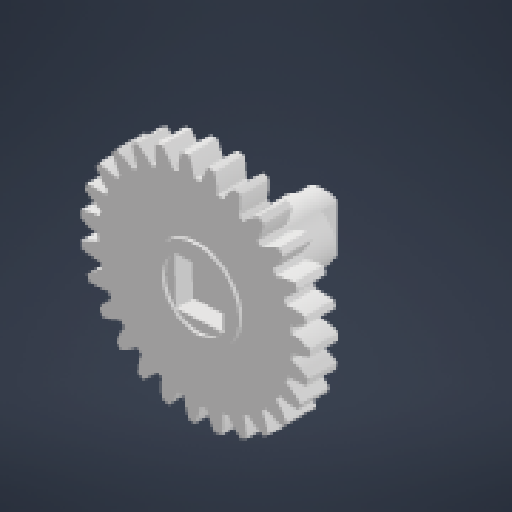
# Autodesk Inventor part: central axel
Saved by Autodesk Inventor 2026 (Build 300175050, 175E)
## iProperties
Created: 2026-03-26
Part Number: central axel
Material: Generic
Document SubType Name: Modeling
Designer: sniel
Density: 1 g/cm^3
Appearance: Default
Author: sniel
Autodesk Inventor part; units mm, degrees
ref_plane "YZ Plane" through (0, 0, 0) normal (1, 0, 0) x (0, 1, 0)
ref_plane "XZ Plane" through (0, 0, 0) normal (0, 1, 0) x (-1, 0, 0)
sketch "Sketch1" plane through (0, 0, 0) normal (0, 0, 1) x (1, 0, 0)
  arc A0 (-2.5, -4.3301) -> (2.5, -4.3301) centre (0, 0) ccw
  line L0 (2.5, 4.3301) -> (2.5, -4.3301)
  arc A1 (2.5, 4.3301) -> (-2.5, 4.3301) centre (0, 0) ccw
  line L1 (-2.5, -4.3301) -> (-2.5, 4.3301)
  line L2 (0, -5) -> (0, -4.75)
  circle A2 centre (0, 0) radius 4.75
  line L3 (-2.5, 0) -> (-2.4, 0)
  line L4 (2.5, 0) -> (2.4, 0)
  line L5 (-2.4, 0) -> (-2.4, -4.3863)
  line L6 (2.4, 0) -> (2.4, -4.3863)
  line L7 (2.4, 0) -> (2.4, 4.3863)
  line L8 (-2.4, 0) -> (-2.4, 4.3863)
  point P0 (0, 0)
  point P1 (-2.4, 4.0991)
  point P2 (-2.4, -4.0991)
  point P3 (2.4, -4.0991)
  point P4 (2.4, 4.0991)
  dimension "d0" = 0.25
  dimension "d1" = 0.1
  dimension "d2" = 0.1
  constraints: 18 end point, 9 point on circle, 4 vertical, 2 centre point, 2 horizontal, 2 midpoint, 1 coincident, 3 other
  measures "d0" distance of L2.start L2.end
  measures "d1" distance of L3.start L3.end
  measures "d2" distance of L4.start L4.end
extrude "Extrusion1" add sketch "Sketch1" along normal blind 3 contours L5 L8 A2 L7 L6
ref_plane "Work Plane1" through (-110.4204, -110.4204, 21.5411) normal (0, 0, -1) x (-0.0508, 0.9987, 0)
sketch "Sketch2" plane through (0, 0, 3) normal (0, 0, 1) x (1, 0, 0)
  circle A0 centre (0, 0) radius 5
  dimension "d5" = 10
  constraints: 1 centre point, 1 coincident
  measures "d5" diameter of A0
extrude "Extrusion2" add sketch "Sketch2" along normal up to surface (18.5411 mm away)
sketch "Sketch3" plane through (0, 0, 21.5411) normal (0, 0, 1) x (1, 0, 0)
  arc A0 (-4.8284, 16.7732) -> (-6.3222, 18.8577) centre (-16.1161, 10.2619) ccw
  arc A1 (-6.3222, 18.8577) -> (-7.4127, 18.4955) centre (-0.6419, -0.0624) ccw
  arc A2 (-7.4127, 18.4955) -> (-7.264, 15.2567) centre (5.5779, 17.4691) ccw
  arc A3 (-7.264, 15.2567) -> (-8.1435, 14.8457) centre (-0.6419, -0.0624) ccw
  arc A4 (-8.1435, 14.8457) -> (-10.5324, 17.0378) centre (-18.0799, 6.415) ccw
  arc A5 (-10.5324, 17.0378) -> (-11.5099, 16.4338) centre (-0.6419, -0.0624) ccw
  arc A6 (-11.5099, 16.4338) -> (-10.6183, 13.3166) centre (1.3672, 18.4309) ccw
  arc A7 (-10.6183, 13.3166) -> (-11.3793, 12.7139) centre (-0.6419, -0.0624) ccw
  arc A8 (-11.3793, 12.7139) -> (-14.2093, 14.296) centre (-19.1036, 2.2189) ccw
  arc A9 (-14.2093, 14.296) -> (-15.0212, 13.4828) centre (-0.6419, -0.0624) ccw
  arc A10 (-15.0212, 13.4828) -> (-13.4348, 10.6552) centre (-2.9518, 18.3958) ccw
  arc A11 (-13.4348, 10.6552) -> (-14.0363, 9.8933) centre (-0.6419, -0.0624) ccw
  arc A12 (-14.0363, 9.8933) -> (-17.1549, 10.7801) centre (-19.1321, -2.1002) ccw
  arc A13 (-17.1549, 10.7801) -> (-17.7574, 9.8016) centre (-0.6419, -0.0624) ccw
  arc A14 (-17.7574, 9.8016) -> (-15.5616, 7.4161) centre (-7.1463, 17.3655) ccw
  arc A15 (-15.5616, 7.4161) -> (-15.9712, 6.5359) centre (-0.6419, -0.0624) ccw
  arc A16 (-15.9712, 6.5359) -> (-19.2102, 6.6796) centre (-18.1638, -6.3094) ccw
  arc A17 (-19.2102, 6.6796) -> (-19.5708, 5.5886) centre (-0.6419, -0.0624) ccw
  arc A18 (-19.5708, 5.5886) -> (-16.8841, 3.7738) centre (-10.9901, 15.3958) ccw
  arc A19 (-16.8841, 3.7738) -> (-17.0797, 2.8229) centre (-0.6419, -0.0624) ccw
  arc A20 (-17.0797, 2.8229) -> (-20.2645, 2.2158) centre (-16.2508, -10.1818) ccw
  arc A21 (-20.2645, 2.2158) -> (-20.3638, 1.0709) centre (-0.6419, -0.0624) ccw
  arc A22 (-20.3638, 1.0709) -> (-17.331, -0.0753) centre (-14.2761, 12.5926) ccw
  arc A23 (-17.331, -0.0753) -> (-17.302, -1.0457) centre (-0.6419, -0.0624) ccw
  arc A24 (-17.302, -1.0457) -> (-20.261, -2.3709) centre (-13.4964, -13.5087) ccw
  arc A25 (-20.261, -2.3709) -> (-20.0936, -3.5078) centre (-0.6419, -0.0624) ccw
  arc A26 (-20.0936, -3.5078) -> (-16.8782, -3.9237) centre (-16.827, 9.1072) ccw
  arc A27 (-16.8782, -3.9237) -> (-16.6262, -4.8613) centre (-0.6419, -0.0624) ccw
  arc A28 (-16.6262, -4.8613) -> (-19.1998, -6.8332) centre (-10.049, -16.1107) ccw
  arc A29 (-19.1998, -6.8332) -> (-18.7747, -7.9008) centre (-0.6419, -0.0624) ccw
  arc A30 (-18.7747, -7.9008) -> (-15.55, -7.564) centre (-18.5054, 5.1275) ccw
  arc A31 (-15.55, -7.564) -> (-15.0886, -8.4181) centre (-0.6419, -0.0624) ccw
  arc A32 (-15.0886, -8.4181) -> (-17.1381, -10.9304) centre (-6.0944, -17.8475) ccw
  arc A33 (-17.1381, -10.9304) -> (-16.4783, -11.8712) centre (-0.6419, -0.0624) ccw
  arc A34 (-16.4783, -11.8712) -> (-13.4182, -10.7998) centre (-19.2208, 0.868) ccw
  arc A35 (-13.4182, -10.7998) -> (-12.7722, -11.5246) centre (-0.6419, -0.0624) ccw
  arc A36 (-12.7722, -11.5246) -> (-14.1871, -14.4418) centre (-1.8459, -18.6256) ccw
  arc A37 (-14.1871, -14.4418) -> (-13.3281, -15.205) centre (-0.6419, -0.0624) ccw
  arc A38 (-13.3281, -15.205) -> (-10.5976, -13.4568) centre (-18.9346, -3.4416) ccw
  arc A39 (-10.5976, -13.4568) -> (-9.8019, -14.013) centre (-0.6419, -0.0624) ccw
  arc A40 (-9.8019, -14.013) -> (-10.5059, -17.1779) centre (2.4675, -18.4029) ccw
  arc A41 (-10.5059, -17.1779) -> (-9.494, -17.7225) centre (-0.6419, -0.0624) ccw
  arc A42 (-9.494, -17.7225) -> (-7.2402, -15.3917) centre (-17.6622, -7.5691) ccw
  arc A43 (-7.2402, -15.3917) -> (-6.3378, -15.7494) centre (-0.6419, -0.0624) ccw
  arc A44 (-6.3378, -15.7494) -> (-6.2929, -18.9913) centre (6.6133, -17.1914) ccw
  arc A45 (-6.2929, -18.9913) -> (-5.1827, -19.2879) centre (-0.6419, -0.0624) ccw
  arc A46 (-5.1827, -19.2879) -> (-3.5272, -16.5002) centre (-15.4722, -11.2919) ccw
  arc A47 (-3.5272, -16.5002) -> (-2.5666, -16.6401) centre (-0.6419, -0.0624) ccw
  arc A48 (-2.5666, -16.6401) -> (-1.7752, -19.7843) centre (10.3679, -15.0565) ccw
  arc A49 (-1.7752, -19.7843) -> (-0.6266, -19.8168) centre (-0.6419, -0.0624) ccw
  arc A50 (-0.6266, -19.8168) -> (0.3414, -16.7225) centre (-12.4828, -14.4093) ccw
  arc A51 (0.3414, -16.7225) -> (1.3084, -16.6371) centre (-0.6419, -0.0624) ccw
  arc A52 (1.3084, -16.6371) -> (2.8035, -19.5141) centre (13.5291, -12.1133) ccw
  arc A53 (2.8035, -19.5141) -> (3.9287, -19.2808) centre (-0.6419, -0.0624) ccw
  arc A54 (3.9287, -19.2808) -> (4.157, -16.0467) centre (-8.8549, -16.7533) ccw
  arc A55 (4.157, -16.0467) -> (5.0782, -15.7406) centre (-0.6419, -0.0624) ccw
  arc A56 (5.0782, -15.7406) -> (7.1965, -18.1952) centre (15.9262, -8.5204) ccw
  arc A57 (7.1965, -18.1952) -> (8.2375, -17.7087) centre (-0.6419, -0.0624) ccw
  arc A58 (8.2375, -17.7087) -> (7.7138, -14.5091) centre (-4.7844, -18.1975) ccw
  arc A59 (7.7138, -14.5091) -> (8.5397, -13.9988) centre (-0.6419, -0.0624) ccw
  arc A60 (8.5397, -13.9988) -> (11.1669, -15.8988) centre (17.4302, -4.4716) ccw
  arc A61 (11.1669, -15.8988) -> (12.0677, -15.1853) centre (-0.6419, -0.0624) ccw
  arc A62 (12.0677, -15.1853) -> (10.8202, -12.1927) centre (-0.4905, -18.664) ccw
  arc A63 (10.8202, -12.1927) -> (11.5062, -11.5058) centre (-0.6419, -0.0624) ccw
  arc A64 (11.5062, -11.5058) -> (14.5007, -12.7486) centre (17.9599, -0.185) ccw
  arc A65 (14.5007, -12.7486) -> (15.2127, -11.8467) centre (-0.6419, -0.0624) ccw
  arc A66 (15.2127, -11.8467) -> (13.3087, -9.2224) centre (3.7952, -18.1276) ccw
  arc A67 (13.3087, -9.2224) -> (13.8177, -8.3958) centre (-0.6419, -0.0624) ccw
  arc A68 (13.8177, -8.3958) -> (17.0182, -8.9145) centre (17.4867, 4.1081) ccw
  arc A69 (17.0182, -8.9145) -> (17.503, -7.8727) centre (-0.6419, -0.0624) ccw
  arc A70 (17.503, -7.8727) -> (15.0451, -5.7583) centre (7.8418, -16.6174) ccw
  arc A71 (15.0451, -5.7583) -> (15.3498, -4.8365) centre (-0.6419, -0.0624) ccw
  arc A72 (15.3498, -4.8365) -> (18.5836, -4.6032) centre (16.0363, 8.1765) ccw
  arc A73 (18.5836, -4.6032) -> (18.8151, -3.4777) centre (-0.6419, -0.0624) ccw
  arc A74 (18.8151, -3.4777) -> (15.9358, -1.9871) centre (11.4309, -14.2147) ccw
  arc A75 (15.9358, -1.9871) -> (16.0197, -1.0199) centre (-0.6419, -0.0624) ccw
  arc A76 (16.0197, -1.0199) -> (19.1125, -0.0471) centre (13.6867, 11.8006) ccw
  arc A77 (19.1125, -0.0471) -> (19.0782, 1.1015) centre (-0.6419, -0.0624) ccw
  arc A78 (19.0782, 1.1015) -> (15.9328, 1.8879) centre (14.3693, -11.049) ccw
  arc A79 (15.9328, 1.8879) -> (15.7914, 2.8483) centre (-0.6419, -0.0624) ccw
  arc A80 (15.7914, 2.8483) -> (18.5765, 4.5082) centre (10.5647, 14.7853) ccw
  arc A81 (18.5765, 4.5082) -> (18.2783, 5.6179) centre (-0.6419, -0.0624) ccw
  arc A82 (18.2783, 5.6179) -> (15.0363, 5.6577) centre (16.4983, -7.2911) ccw
  arc A83 (15.0363, 5.6577) -> (14.6772, 6.5597) centre (-0.6419, -0.0624) ccw
  arc A84 (14.6772, 6.5597) -> (17.0044, 8.817) centre (6.8385, 16.9695) ccw
  arc A85 (17.0044, 8.817) -> (16.4583, 9.8281) centre (-0.6419, -0.0624) ccw
  arc A86 (16.4583, 9.8281) -> (13.2945, 9.1192) centre (17.7033, -3.1434) ccw
  arc A87 (13.2945, 9.1192) -> (12.7371, 9.914) centre (-0.6419, -0.0624) ccw
  arc A88 (12.7371, 9.914) -> (14.481, 12.6472) centre (2.709, 18.2355) ccw
  arc A89 (14.481, 12.6472) -> (13.7165, 13.505) centre (-0.6419, -0.0624) ccw
  arc A90 (13.7165, 13.505) -> (10.8014, 12.0857) centre (17.9194, 1.1703) ccw
  arc A91 (10.8014, 12.0857) -> (10.0757, 12.7305) centre (-0.6419, -0.0624) ccw
  arc A92 (10.0757, 12.7305) -> (11.1424, 15.7922) centre (-1.6011, 18.515) ccw
  arc A93 (11.1424, 15.7922) -> (10.2006, 16.4506) centre (-0.6419, -0.0624) ccw
  arc A94 (10.2006, 16.4506) -> (7.6915, 14.3972) centre (17.1348, 5.4176) ccw
  arc A95 (7.6915, 14.3972) -> (6.8366, 14.8573) centre (-0.6419, -0.0624) ccw
  arc A96 (6.8366, 14.8573) -> (7.1684, 18.0825) centre (-5.8595, 17.793) ccw
  arc A97 (7.1684, 18.0825) -> (6.1001, 18.5059) centre (-0.6419, -0.0624) ccw
  arc A98 (6.1001, 18.5059) -> (4.1322, 15.9293) centre (15.3918, 9.3695) ccw
  arc A99 (4.1322, 15.9293) -> (3.1943, 16.1798) centre (-0.6419, -0.0624) ccw
  arc A100 (3.1943, 16.1798) -> (2.7734, 19.3946) centre (-9.8366, 16.1085) ccw
  arc A101 (2.7734, 19.3946) -> (1.6363, 19.5602) centre (-0.6419, -0.0624) ccw
  arc A102 (1.6363, 19.5602) -> (0.5307, 17.2462) centre (12.7845, 12.8129) ccw
  arc A103 (0.5307, 17.2462) -> (0.5011, 17.1057) centre (20.0615, 13.0592) ccw
  arc A104 (0.5011, 17.1057) -> (0.4804, 17.1045) centre (5.7469, -72.441) ccw
  arc A105 (0.4804, 17.1045) -> (0.3156, 16.5992) centre (12.7845, 12.8129) ccw
  arc A106 (0.3156, 16.5992) -> (-0.6548, 16.6267) centre (-0.6419, -0.0624) ccw
  arc A107 (-0.6548, 16.6267) -> (-1.8058, 19.6577) centre (-13.318, 13.5522) ccw
  arc A108 (-1.8058, 19.6577) -> (-2.9504, 19.5567) centre (-0.6419, -0.0624) ccw
  arc A109 (-2.9504, 19.5567) -> (-3.5527, 16.3709) centre (9.4533, 15.5622) ccw
  arc A110 (-3.5527, 16.3709) -> (-4.5032, 16.1738) centre (-0.6419, -0.0624) ccw
  arc A111 (-4.5032, 16.1738) -> (-4.754, 16.6425) centre (-16.1161, 10.2619) ccw
  arc A112 (-4.754, 16.6425) -> (-4.7746, 16.64) centre (5.7469, -72.441) ccw
  arc A113 (-4.7746, 16.64) -> (-4.8284, 16.7732) centre (-23.3238, 9.2297) ccw
  point P0 (0, 0)
  constraints: 228 point on circle, 114 centre point
extrude "Extrusion3" add sketch "Sketch3" against normal blind 5
sketch "Sketch4" plane through (5.5779, 17.4691, 21.5411) normal (0, 0, 1) x (0.9989, 0.0459, 0)
  circle A0 centre (-6.3733, -17.1949) radius 5.75
  line L0 (-6.3733, -17.1949) -> (-2.3074, -21.2608)
  line L1 (-6.3733, -17.1949) -> (-0.6233, -17.1949) construction
  line L2 (-10.4392, -13.129) -> (-2.3074, -13.129)
  line L3 (-2.3074, -13.129) -> (-2.3074, -21.2608)
  line L4 (-2.3074, -21.2608) -> (-10.4392, -21.2608)
  line L5 (-10.4392, -21.2608) -> (-10.4392, -13.129)
  line L6 (-10.4392, -13.129) -> (-2.3074, -21.2608) construction
  line L7 (-2.3074, -13.129) -> (-10.4392, -21.2608) construction
  arc A1 (-6.4028, -11.181) -> (-6.3438, -23.2088) centre (-6.3733, -17.1949) ccw projected
  point P0 (-6.3733, -17.1949)
  dimension "d10" = 11.5
  dimension "d11" = 45
  constraints: 16 end point, 2 horizontal, 2 midpoint, 2 parallel, 1 equal length, 1 perpendicular, 3 other
  measures "d11" angle of L0 L1
extrude "Extrusion4" cut sketch "Sketch4" against normal blind 3 contours L3 L4 L5 L2
sketch "Sketch5" plane through (5.5779, 17.4691, 21.5411) normal (0, 0, 1) x (0.9989, 0.0459, 0)
  line L0 (-2.3074, -13.129) -> (-2.3074, -21.2608) projected
  line L1 (-2.3074, -21.2608) -> (-10.4392, -21.2608) projected
  line L2 (-10.4392, -21.2608) -> (-10.4392, -13.129) projected
  line L3 (-10.4392, -13.129) -> (-2.3074, -13.129) projected
  arc A0 (-11.8239, 1.933) -> (-12.9299, 1.6211) centre (-7.0174, -17.2278) ccw projected
  arc A1 (-12.9299, 1.6211) -> (-12.9299, -1.6211) centre (0, 0) ccw projected
  arc A2 (-12.9299, -1.6211) -> (-13.8273, -1.9913) centre (-7.0174, -17.2278) ccw projected
  arc A3 (-13.8273, -1.9913) -> (-16.1131, 0.3081) centre (-24.1399, -9.9574) ccw projected
  arc A4 (-16.1131, 0.3081) -> (-17.1173, -0.2505) centre (-7.0174, -17.2278) ccw projected
  arc A5 (-17.1173, -0.2505) -> (-16.3696, -3.4053) centre (-4.1622, 1.1539) ccw projected
  arc A6 (-16.3696, -3.4053) -> (-17.1575, -3.9725) centre (-7.0174, -17.2278) ccw projected
  arc A7 (-17.1575, -3.9725) -> (-19.912, -2.2622) centre (-25.3551, -14.1021) ccw projected
  arc A8 (-19.912, -2.2622) -> (-20.7603, -3.0373) centre (-7.0174, -17.2278) ccw projected
  arc A9 (-20.7603, -3.0373) -> (-19.3052, -5.9347) centre (-8.4782, 1.3169) ccw projected
  arc A10 (-19.3052, -5.9347) -> (-19.9411, -6.6682) centre (-7.0174, -17.2278) ccw projected
  arc A11 (-19.9411, -6.6682) -> (-23.0157, -5.6393) centre (-25.5816, -18.4153) ccw projected
  arc A12 (-23.0157, -5.6393) -> (-23.6624, -6.5892) centre (-7.0174, -17.2278) ccw projected
  arc A13 (-23.6624, -6.5892) -> (-21.5784, -9.0728) centre (-12.7156, 0.4802) ccw projected
  arc A14 (-21.5784, -9.0728) -> (-22.0279, -9.9333) centre (-7.0174, -17.2278) ccw projected
  arc A15 (-22.0279, -9.9333) -> (-25.2569, -9.6412) centre (-24.8074, -22.6645) ccw projected
  arc A16 (-25.2569, -9.6412) -> (-25.6672, -10.7145) centre (-7.0174, -17.2278) ccw projected
  arc A17 (-25.6672, -10.7145) -> (-23.0666, -12.6506) centre (-16.6457, -1.3113) ccw projected
  arc A18 (-23.0666, -12.6506) -> (-23.3055, -13.5916) centre (-7.0174, -17.2278) ccw projected
  arc A19 (-23.3055, -13.5916) -> (-26.5149, -14.052) centre (-23.074, -26.6206) ccw projected
  arc A20 (-26.5149, -14.052) -> (-26.6666, -15.191) centre (-7.0174, -17.2278) ccw projected
  arc A21 (-26.6666, -15.191) -> (-23.6895, -16.4752) centre (-20.0568, -3.9607) ccw projected
  arc A22 (-23.6895, -16.4752) -> (-23.7051, -17.4459) centre (-7.0174, -17.2278) ccw projected
  arc A23 (-23.7051, -17.4459) -> (-26.7217, -18.634) centre (-20.4751, -30.0703) ccw projected
  arc A24 (-26.7217, -18.634) -> (-26.6066, -19.7774) centre (-7.0174, -17.2278) ccw projected
  arc A25 (-26.6066, -19.7774) -> (-23.4137, -20.3404) centre (-22.7649, -7.3254) ccw projected
  arc A26 (-23.4137, -20.3404) -> (-23.2049, -21.2884) centre (-7.0174, -17.2278) ccw projected
  arc A27 (-23.2049, -21.2884) -> (-25.8663, -23.1402) centre (-17.1506, -32.8277) ccw projected
  arc A28 (-25.8663, -23.1402) -> (-25.4906, -24.2262) centre (-7.0174, -17.2278) ccw projected
  arc A29 (-25.4906, -24.2262) -> (-22.2539, -24.0377) centre (-24.6241, -11.224) ccw projected
  arc A30 (-22.2539, -24.0377) -> (-21.8322, -24.9121) centre (-7.0174, -17.2278) ccw projected
  arc A31 (-21.8322, -24.9121) -> (-23.9947, -27.3277) centre (-13.2799, -34.7441) ccw projected
  arc A32 (-23.9947, -27.3277) -> (-23.3787, -28.2978) centre (-7.0174, -17.2278) ccw projected
  arc A33 (-23.3787, -28.2978) -> (-20.2727, -27.3679) centre (-25.534, -15.4462) ccw projected
  arc A34 (-20.2727, -27.3679) -> (-19.6607, -28.1215) centre (-7.0174, -17.2278) ccw projected
  arc A35 (-19.6607, -28.1215) -> (-21.2079, -30.9707) centre (-9.0716, -35.7162) ccw projected
  arc A36 (-21.2079, -30.9707) -> (-20.3848, -31.7726) centre (-7.0174, -17.2278) ccw projected
  arc A37 (-20.3848, -31.7726) -> (-17.5769, -30.1515) centre (-25.4458, -19.7644) ccw projected
  arc A38 (-17.5769, -30.1515) -> (-16.8076, -30.7436) centre (-7.0174, -17.2278) ccw projected
  arc A39 (-16.8076, -30.7436) -> (-17.656, -33.8728) centre (-4.7525, -35.6916) ccw projected
  arc A40 (-17.656, -33.8728) -> (-16.6702, -34.4632) centre (-7.0174, -17.2278) ccw projected
  arc A41 (-16.6702, -34.4632) -> (-14.3119, -32.2383) centre (-24.3641, -23.9459) ccw projected
  arc A42 (-14.3119, -32.2383) -> (-13.4268, -32.6371) centre (-7.0174, -17.2278) ccw projected
  arc A43 (-13.4268, -32.6371) -> (-13.5306, -35.8776) centre (-0.5555, -34.6715) ccw projected
  arc A44 (-13.5306, -35.8776) -> (-12.4352, -36.2248) centre (-7.0174, -17.2278) ccw projected
  arc A45 (-12.4352, -36.2248) -> (-10.6536, -33.5159) centre (-22.3472, -27.7653) ccw projected
  arc A46 (-10.6536, -33.5159) -> (-9.7004, -33.6998) centre (-7.0174, -17.2278) ccw projected
  arc A47 (-9.7004, -33.6998) -> (-9.0541, -36.8769) centre (3.2931, -32.7111) ccw projected
  arc A48 (-9.0541, -36.8769) -> (-7.9082, -36.9621) centre (-7.0174, -17.2278) ccw projected
  arc A49 (-7.9082, -36.9621) -> (-6.7993, -33.9155) centre (-19.5038, -31.0165) ccw projected
  arc A50 (-6.7993, -33.9155) -> (-5.8294, -33.8745) centre (-7.0174, -17.2278) ccw projected
  arc A51 (-5.8294, -33.8745) -> (-4.4678, -36.817) centre (6.5859, -29.916) ccw projected
  arc A52 (-4.4678, -36.817) -> (-3.3331, -36.6356) centre (-7.0174, -17.2278) ccw projected
  arc A53 (-3.3331, -36.6356) -> (-2.9567, -33.4153) centre (-15.9874, -33.5244) ccw projected
  arc A54 (-2.9567, -33.4153) -> (-2.0224, -33.1518) centre (-7.0174, -17.2278) ccw projected
  arc A55 (-2.0224, -33.1518) -> (-0.019, -35.701) centre (9.1453, -26.4368) ccw projected
  arc A56 (-0.019, -35.701) -> (1.0433, -35.2628) centre (-7.0174, -17.2278) ccw projected
  arc A57 (1.0433, -35.2628) -> (0.6669, -32.0426) centre (-11.9873, -35.1538) ccw projected
  arc A58 (0.6669, -32.0426) -> (1.5153, -31.5707) centre (-7.0174, -17.2278) ccw projected
  arc A59 (1.5153, -31.5707) -> (4.0526, -33.5891) centre (10.8334, -22.4612) ccw projected
  arc A60 (4.0526, -33.5891) -> (4.9852, -32.9178) centre (-7.0174, -17.2278) ccw projected
  arc A61 (4.9852, -32.9178) -> (3.8763, -29.8711) centre (-7.7193, -35.8167) ccw projected
  arc A62 (3.8763, -29.8711) -> (4.593, -29.2163) centre (-7.0174, -17.2278) ccw projected
  arc A63 (4.593, -29.2163) -> (7.5274, -30.5952) centre (11.5592, -18.2035) ccw projected
  arc A64 (7.5274, -30.5952) -> (8.28, -29.7269) centre (-7.0174, -17.2278) ccw projected
  arc A65 (8.28, -29.7269) -> (6.4984, -27.018) centre (-3.4135, -35.4775) ccw projected
  arc A66 (6.4984, -27.018) -> (7.0448, -26.2156) centre (-7.0174, -17.2278) ccw projected
  arc A67 (7.0448, -26.2156) -> (10.2181, -26.8806) centre (11.2834, -13.8931) ccw projected
  arc A68 (10.2181, -26.8806) -> (10.7502, -25.8621) centre (-7.0174, -17.2278) ccw projected
  arc A69 (10.7502, -25.8621) -> (8.3919, -23.6372) centre (0.698, -34.1545) ccw projected
  arc A70 (8.3919, -23.6372) -> (8.7385, -22.7304) centre (-7.0174, -17.2278) ccw projected
  arc A71 (8.7385, -22.7304) -> (11.9796, -22.6456) centre (10.0211, -9.7626) ccw projected
  arc A72 (11.9796, -22.6456) -> (12.2625, -21.5319) centre (-7.0174, -17.2278) ccw projected
  arc A73 (12.2625, -21.5319) -> (9.4546, -19.9108) centre (4.3936, -31.9189) ccw projected
  arc A74 (9.4546, -19.9108) -> (9.5828, -18.9485) centre (-7.0174, -17.2278) ccw projected
  arc A75 (9.5828, -18.9485) -> (12.7169, -18.1186) centre (7.8402, -6.0344) ccw projected
  arc A76 (12.7169, -18.1186) -> (12.7354, -16.9696) centre (-7.0174, -17.2278) ccw projected
  arc A77 (12.7354, -16.9696) -> (9.6294, -16.0398) centre (7.474, -28.8914) ccw projected
  arc A78 (9.6294, -16.0398) -> (9.5321, -15.0738) centre (-7.0174, -17.2278) ccw projected
  arc A79 (9.5321, -15.0738) -> (12.3904, -13.5435) centre (4.8584, -2.9097) ccw projected
  arc A80 (12.3904, -13.5435) -> (12.1434, -12.4213) centre (-7.0174, -17.2278) ccw projected
  arc A81 (12.1434, -12.4213) -> (8.9067, -12.2328) centre (9.7732, -25.235) ccw projected
  arc A82 (8.9067, -12.2328) -> (8.5893, -11.3153) centre (-7.0174, -17.2278) ccw projected
  arc A83 (8.5893, -11.3153) -> (11.0177, -9.1671) centre (1.2363, -0.5569) ccw projected
  arc A84 (11.0177, -9.1671) -> (10.5184, -8.1321) centre (-7.0174, -17.2278) ccw projected
  arc A85 (10.5184, -8.1321) -> (7.3255, -8.6951) centre (11.1672, -21.147) ccw projected
  arc A86 (7.3255, -8.6951) -> (6.8051, -7.8755) centre (-7.0174, -17.2278) ccw projected
  arc A87 (6.8051, -7.8755) -> (8.6726, -5.2252) centre (-2.8307, 0.8971) ccw projected
  arc A88 (8.6726, -5.2252) -> (7.9482, -4.3332) centre (-7.0174, -17.2278) ccw projected
  arc A89 (7.9482, -4.3332) -> (4.9711, -5.6174) centre (11.5809, -16.8477) ccw projected
  arc A90 (4.9711, -5.6174) -> (4.2757, -4.94) centre (-7.0174, -17.2278) ccw projected
  arc A91 (4.2757, -4.94) -> (5.4817, -1.9304) centre (-7.1235, 1.3741) ccw projected
  arc A92 (5.4817, -1.9304) -> (4.5711, -1.2295) centre (-7.0174, -17.2278) ccw projected
  arc A93 (4.5711, -1.2295) -> (1.9704, -3.1656) centre (10.9919, -12.5689) ccw projected
  arc A94 (1.9704, -3.1656) -> (1.1376, -2.6668) centre (-7.0174, -17.2278) ccw projected
  arc A95 (1.1376, -2.6668) -> (1.6169, 0.5398) centre (-11.4105, 0.8482) ccw projected
  arc A96 (1.6169, 0.5398) -> (0.5692, 1.0118) centre (-7.0174, -17.2278) ccw projected
  arc A97 (0.5692, 1.0118) -> (-1.5148, -1.4719) centre (9.432, -8.5412) ccw projected
  arc A98 (-1.5148, -1.4719) -> (-2.4402, -1.1786) centre (-7.0174, -17.2278) ccw projected
  arc A99 (-2.4402, -1.1786) -> (-2.7133, 2.0521) centre (-15.4607, -0.6522) ccw projected
  arc A100 (-2.7133, 2.0521) -> (-3.8416, 2.2697) centre (-7.0174, -17.2278) ccw projected
  arc A101 (-3.8416, 2.2697) -> (-5.0521, 0.0088) centre (6.9854, -4.9819) ccw projected
  arc A102 (-5.0521, 0.0088) -> (-5.0881, -0.1301) centre (14.2661, -5.0696) ccw projected
  arc A103 (-5.0881, -0.1301) -> (-5.1089, -0.1304) centre (-3.9551, -89.8232) ccw projected
  arc A104 (-5.1089, -0.1304) -> (-5.2967, -0.6276) centre (6.9854, -4.9819) ccw projected
  arc A105 (-5.2967, -0.6276) -> (-6.2648, -0.5557) centre (-7.0174, -17.2278) ccw projected
  arc A106 (-6.2648, -0.5557) -> (-7.2755, 2.525) centre (-19.0557, -3.0461) ccw projected
  arc A107 (-7.2755, 2.525) -> (-8.4236, 2.4765) centre (-7.0174, -17.2278) ccw projected
  arc A108 (-8.4236, 2.4765) -> (-9.1713, -0.6783) centre (3.7838, -2.0827) ccw projected
  arc A109 (-9.1713, -0.6783) -> (-10.13, -0.8315) centre (-7.0174, -17.2278) ccw projected
  arc A110 (-10.13, -0.8315) -> (-10.3589, -0.3519) centre (-22.0017, -6.2046) ccw projected
  arc A111 (-10.3589, -0.3519) -> (-10.3797, -0.3534) centre (-3.9551, -89.8232) ccw projected
  arc A112 (-10.3797, -0.3534) -> (-10.4273, -0.2179) centre (-29.2492, -6.9051) ccw projected
  arc A113 (-10.4273, -0.2179) -> (-11.8239, 1.933) centre (-22.0017, -6.2046) ccw projected
  circle A114 centre (-6.3733, -17.1949) radius 5.75 projected
  circle A115 centre (-6.3733, -17.1949) radius 7.5
  point P0 (-6.3733, -17.1949)
  dimension "d14" = 15
  constraints: 1 centre point, 1 coincident
  measures "d14" diameter of A115
extrude "Extrusion5" add sketch "Sketch5" along normal blind 0.58 contours A115
body "Solid1"
